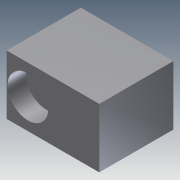
# Autodesk Inventor part: basic1
Saved by Autodesk Inventor 2011 (Build 150239000, 239)
## iProperties
Created: 2011-12-10
Part Number: basic1
Document SubType Name: Modeling
Designer: Matthew
Density: 1 g/cm^3
Author: Matthew
Autodesk Inventor part; units mm, degrees
ref_plane "YZ Plane" through (0, 0, 0) normal (1, 0, 0) x (0, 1, 0)
ref_plane "XZ Plane" through (0, 0, 0) normal (0, 1, 0) x (-1, 0, 0)
ref_plane "XY Plane" through (0, 0, 0) normal (0, 0, 1) x (1, 0, 0)
sketch "Sketch1" plane through (0, 0, 0) normal (0, 0, 1) x (1, 0, 0)
  line L0 (-20.1009, 13.5086) -> (29.8991, 13.5086)
  line L1 (29.8991, 13.5086) -> (29.8991, -18.4914)
  line L2 (29.8991, -18.4914) -> (-20.1009, -18.4914)
  line L3 (-20.1009, -18.4914) -> (-20.1009, 13.5086)
  point P0 (0, 0)
  dimension "d0" = 50
  dimension "d1" = 32
  constraints: 8 end point, 2 parallel, 1 horizontal, 1 perpendicular
  measures "d0" distance of L0.end L0.start
  measures "d1" distance of L2.end L0.start
extrude "Extrusion1" add sketch "Sketch1" along normal blind 40
sketch "Sketch2" plane through (0, 0, 40) normal (0, 0, 1) x (1, 0, 0)
  line L0 (-20.1009, -18.4914) -> (-20.1009, 13.5086) projected
  line L1 (29.8991, -18.4914) -> (-20.1009, -18.4914) projected
  line L2 (-20.1009, -2.4914) -> (-8.6009, -2.4914)
  circle A0 centre (-8.6009, -2.4914) radius 8
  point P0 (0, 0)
  dimension "d4" = 11.5
  dimension "d5" = 16
  constraints: 2 end point, 1 centre point, 1 coincident, 1 midpoint, 1 parallel
  measures "d4" distance of L2.start L2.end
  measures "d5" diameter of A0
extrude "Extrusion2" cut sketch "Sketch2" against normal blind 10
sketch "Sketch3" plane through (0, 0, 40) normal (0, 0, 1) x (1, 0, 0)
  circle A0 centre (-8.6009, -2.4914) radius 8 projected
  point P0 (0, 0)
extrude "Extrusion3" add sketch "Sketch3" against normal blind 10
sketch "Sketch4" plane through (0, 0, 40) normal (0, 0, 1) x (1, 0, 0)
  line L0 (-20.1009, -18.4914) -> (-20.1009, 13.5086) projected
  line L1 (29.8991, -18.4914) -> (-20.1009, -18.4914) projected
  line L2 (-20.1009, -2.4914) -> (-8.6009, -2.4914)
  circle A0 centre (-8.6009, -2.4914) radius 11
  point P0 (0, 0)
  dimension "d10" = 11.5
  dimension "d11" = 22
  constraints: 2 end point, 1 centre point, 1 coincident, 1 midpoint, 1 parallel
  measures "d10" distance of L2.start L2.end
  measures "d11" diameter of A0
extrude "Extrusion4" cut sketch "Sketch4" against normal blind 10
body "Solid1"
